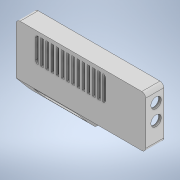
# Autodesk Inventor part: top
Saved by Autodesk Inventor 2021 (Build 250183000, 183)
## iProperties
Created: 2024-09-17
Part Number: top
Material: Generic
Document SubType Name: Modeling
Designer: Toby
Density: 1 g/cm^3
Appearance: Default
Author: Toby
Autodesk Inventor part; units mm, degrees
ref_plane "YZ Plane" through (0, 0, 0) normal (1, 0, 0) x (0, 1, 0)
ref_plane "XZ Plane" through (0, 0, 0) normal (0, 1, 0) x (-1, 0, 0)
ref_plane "XY Plane" through (0, 0, 0) normal (0, 0, 1) x (1, 0, 0)
sketch "Sketch1" plane through (0, 0, 0) normal (0, 0, 1) x (1, 0, 0)
  line L0 (-50, 26) -> (50, 26)
  line L1 (50, 26) -> (50, -26)
  line L2 (50, -26) -> (-50, -26)
  line L3 (-50, -26) -> (-50, 26)
  point P0 (0, 0)
  dimension "d0" = 52
  dimension "d1" = 100
  dimension "d2" = 26
  dimension "d3" = 50
  constraints: 8 end point, 2 parallel, 1 horizontal, 1 perpendicular
  measures "d0" distance of L2.end L0.start
  measures "d1" distance of L0.start L0.end
  measures "d2" distance from line of point (0, 0) L0
  measures "d3" distance from line of point (0, 0) L3
extrude "Extrusion1" add sketch "Sketch1" along normal blind 2
sketch "Sketch4" plane through (0, 0, 2) normal (0, 0, 1) x (1, 0, 0)
  line L0 (50, -26) -> (50, 26) projected
  line L1 (50, -26) -> (13.1, -26)
  line L2 (13.1, -26) -> (13.1, -13.5)
  line L3 (13.1, -13.5) -> (50, -13.5)
  line L4 (50, -13.5) -> (50, -26)
  line L5 (-50, 26) -> (-50, -26) projected
  point P0 (0, 0)
  dimension "d35" = 12.5
  dimension "d36" = 63.1
  constraints: 8 end point, 2 parallel, 1 horizontal, 1 perpendicular
  measures "d35" distance between parallel lines of L1 L3
  measures "d36" distance between parallel lines of L5 L2
extrude "Extrusion3" cut sketch "Sketch4" against normal blind 3
sketch "Sketch5" plane through (0, 0, 2) normal (0, 0, 1) x (1, 0, 0)
  line L0 (-50, -26) -> (13.1, -26) projected
  line L1 (-50, 26) -> (-50, -26) projected
  line L2 (13.1, -13.5) -> (0.673, -26)
  line L3 (0.673, -26) -> (13.1, -26)
  line L4 (13.1, -26) -> (13.1, -13.5) projected
  line L5 (13.1, -13.5) -> (13.1, -26)
  point P0 (0, 0)
  dimension "d39" = 50.673
  constraints: 6 end point, 1 horizontal, 1 point on line, 1 vertical
  measures "d39" distance from line of L1 L2.end
extrude "Extrusion4" cut sketch "Sketch5" against normal blind 3
sketch "Sketch13" plane through (0, 0, 0) normal (0, 0, -1) x (-1, 0, 0)
  line L0 (50, 26) -> (50, -26) projected
  line L1 (-50, 26) -> (50, 26) projected
  line L2 (50, -26) -> (48, -26)
  line L3 (48, -26) -> (48, 26)
  line L4 (48, 26) -> (50, 26)
  line L5 (50, 26) -> (50, -26)
  line L6 (48, 26) -> (-50, 26)
  line L7 (-50, 26) -> (-50, 24)
  line L8 (-50, 24) -> (48, 24)
  line L9 (48, 24) -> (48, 26)
  line L10 (-50, -13.5) -> (-50, 26) projected
  line L11 (-50, -13.5) -> (-48, -13.5)
  line L12 (-48, -13.5) -> (-48, 24)
  line L13 (-48, 24) -> (-50, 24)
  line L14 (-50, 24) -> (-50, -13.5)
  line L15 (6, 24) -> (-9, 24)
  line L16 (-9, 24) -> (-9, 24.8)
  line L17 (-9, 24.8) -> (6, 24.8)
  line L18 (6, 24.8) -> (6, 24)
  point P0 (0, 0)
  dimension "d79" = 2
  dimension "d80" = 2
  dimension "d81" = 2
  dimension "d82" = 1.2
  dimension "d83" = 44
  dimension "d84" = 59
  constraints: 32 end point, 8 parallel, 4 horizontal, 4 perpendicular, 3 point on line, 1 collinear
  measures "d79" distance of L3.end L4.end
  measures "d80" distance between parallel lines of L1 L8
  measures "d81" distance between parallel lines of L10 L12
  measures "d82" distance between parallel lines of L6 L17
  measures "d83" distance between parallel lines of L0 L18
  measures "d84" distance between parallel lines of L0 L16
extrude "Extrusion12" add sketch "Sketch13" along normal blind 12 contours L0 L2 L3 L1 | L3 L8 L18 L17 L16 L7 L1 | L8 L12 L11 L10
sketch "Sketch14" plane through (0, 0, 0) normal (0, 0, -1) x (-1, 0, 0)
  line L0 (48, -26) -> (48, 24) projected
  line L1 (48, -26) -> (37.4, -26)
  line L2 (37.4, -26) -> (37.4, -24)
  line L3 (37.4, -24) -> (48, -24)
  line L4 (48, -24) -> (48, -26)
  line L5 (50, -26) -> (50, 26) projected
  point P0 (0, 0)
  dimension "d87" = 2
  dimension "d88" = 12.6
  constraints: 8 end point, 2 parallel, 1 horizontal, 1 perpendicular
  measures "d87" distance between parallel lines of L1 L3
  measures "d88" distance between parallel lines of L5 L2
extrude "Extrusion13" add sketch "Sketch14" along normal blind 12
fillet "Fillet3" radius 3 4 edges at (-50, -26, -5) (-50, 26, -5) (50, 26, -5) (50, -13.5, -5)
sketch "Sketch16" plane through (0, 0, 0) normal (0, 0, -1) x (-1, 0, 0)
  line L0 (37.4, -26) -> (37.4, -24) projected
  line L1 (37.4, -26) -> (-0.673, -26) projected
  line L2 (37.4, -24) -> (3.6, -24)
  line L3 (3.6, -24) -> (3.6, -26)
  line L4 (3.6, -26) -> (37.4, -26)
  line L5 (37.4, -26) -> (37.4, -24)
  point P0 (0, 0)
  dimension "d95" = 33.8
  constraints: 8 end point, 2 parallel, 1 horizontal, 1 perpendicular, 1 point on line
  measures "d95" distance of L0.end L2.end
extrude "Extrusion15" add sketch "Sketch16" along normal blind 4.4
sketch "Sketch21" plane through (0, 0, 0) normal (0, 0, -1) x (-1, 0, 0)
  line L0 (-13.1, -13.5) -> (-0.673, -26) projected
  line L1 (-13.1, -13.5) -> (-0.673, -26)
  line L2 (3.6, -26) -> (3.6, -24) projected
  line L3 (-0.673, -26) -> (3.6, -26)
  line L4 (3.6, -26) -> (3.6, -24)
  line L5 (3.6, -24) -> (-0.673, -24)
  line L6 (-0.673, -24) -> (-13.1, -11.5)
  line L7 (-13.1, -11.5) -> (-13.1, -13.5)
  point P0 (0, 0)
  dimension "d117" = 2
  dimension "d118" = 2
  constraints: 12 end point, 3 equal length, 3 perpendicular
  measures "d117" distance of L2.start L2.end
  measures "d118" distance of L6.end L0.start
extrude "Extrusion20" add sketch "Sketch21" along normal blind 12
sketch "Sketch22" plane through (0, 0, 0) normal (0, 0, -1) x (-1, 0, 0)
  line L0 (-0.673, -24) -> (-13.1, -11.5) projected
  line L1 (-13.1, -13.5) -> (-47, -13.5) projected
  line L2 (-13.1, -11.5) -> (-47, -11.5)
  line L3 (-47, -11.5) -> (-47, -13.5)
  line L4 (-47, -13.5) -> (-13.1, -13.5)
  line L5 (-13.1, -13.5) -> (-13.1, -11.5)
  arc A0 (-48, -13.3284) -> (-47, -13.5) centre (-47, -10.5) ccw projected
  circle A1 centre (-47, -10.5) radius 3
  circle A2 centre (-47, -10.5) radius 1
  line L6 (-48, 24) -> (-48, -13.3284) projected
  line L7 (-48, -10.5) -> (-48, -13.3284)
  line L8 (-48, -13.3284) -> (-47, -13.5)
  point P0 (0, 0)
  constraints: 12 end point, 2 centre point, 2 coincident, 2 parallel, 2 point on circle, 1 collinear, 1 horizontal, 1 perpendicular, 1 point on line, 1 tangent
extrude "Extrusion21" add sketch "Sketch22" along normal blind 12 contours L1 A1 L2 L5 | L8 L6 A2 L3 | L3 L2 A1 | A0 L8
sketch "Sketch23" plane through (13.1, -13.5, -12) normal (0, -1, 0) x (1, 0, 0)
  line L0 (-63.1, 14) -> (-63.1, 0) projected
  circle A0 centre (6.9, 6.7088) radius 4
  circle A1 centre (25.9, 6.7088) radius 4
  line L1 (34.9, 0) -> (-4.1, 0) projected
  line L2 (2.9, 6.7088) -> (10.9, 6.7088)
  line L3 (10.9, 6.7088) -> (10.9, 0)
  line L4 (10.9, 0) -> (2.9, 0)
  line L5 (2.9, 0) -> (2.9, 6.7088)
  line L6 (21.9, 6.7088) -> (29.9, 6.7088)
  line L7 (29.9, 6.7088) -> (29.9, 0)
  line L8 (29.9, 0) -> (21.9, 0)
  line L9 (21.9, 0) -> (21.9, 6.7088)
  point P0 (-13.1, 12)
  point P1 (21.9, 0)
  point P2 (29.9, 6.7088)
  point P3 (2.9, 0)
  dimension "d125" = 8
  dimension "d126" = 8
  dimension "d123" = 70
  dimension "d124" = 89
  constraints: 16 end point, 4 parallel, 3 point on line, 2 coincident, 2 horizontal, 2 perpendicular, 6 other
  measures "d123" distance from line of L0 point (6.9, 6.709)
  measures "d124" distance from line of L0 point (25.9, 6.709)
extrude "Extrusion22" cut sketch "Sketch23" against normal blind 2
sketch "Sketch24" plane through (50, -10.5, -12) normal (1, 0, 0) x (0, 0, -1)
  line L0 (-14, 0) -> (-14, 33.5) projected
  line L1 (0, 36.5) -> (-14, 36.5) projected
  circle A0 centre (-6, 26.5) radius 4
  circle A1 centre (-6, 14.5) radius 4
  point P0 (-12, 10.5)
  dimension "d129" = 8
  dimension "d130" = 10
  dimension "d131" = 12
  dimension "d132" = 8
  dimension "d133" = 8
  dimension "d134" = 8
  constraints: 2 centre point, 2 coincident
  measures "d129" distance from line of point (-6, 26.5) L0
  measures "d130" distance from line of L1 point (-6, 26.5)
  measures "d131" distance of point (-6, 26.5) point (-6, 14.5)
  measures "d132" distance from line of L0 point (-6, 14.5)
  measures "d133" diameter of A0
  measures "d134" diameter of A1
extrude "Extrusion23" cut sketch "Sketch24" against normal blind 2
sketch "Sketch27" plane through (0, 0, -12) normal (0, 0, -1) x (-1, 0, 0)
  line L0 (50, -23) -> (50, 23) projected
  line L1 (-0.673, -26) -> (47, -26) projected
  line L2 (-0.673, -26) -> (3.6, -26) projected
  line L3 (3.6, -26) -> (37.4, -26) projected
  line L4 (47, 26) -> (-47, 26) projected
  circle A0 centre (-47, 23) radius 2.4
  circle A1 centre (-47, -11) radius 2.4
  circle A2 centre (47, -23) radius 2.4
  circle A3 centre (0, -23) radius 2.4
  circle A4 centre (47, 23) radius 2.4
  point P0 (0, 0)
  point P1 (42.2, -26)
  point P2 (5.6, -26)
  dimension "d144" = 3
  dimension "d145" = 3
  dimension "d146" = 3
  dimension "d147" = 50
  dimension "d148" = 97
  dimension "d149" = 15
  dimension "d150" = 3
  dimension "d151" = 3
  dimension "d152" = 97
  dimension "d153" = 49
  dimension "d154" = 4.8
  dimension "d155" = 4.8
  dimension "d156" = 4.8
  dimension "d157" = 4.8
  dimension "d158" = 4.8
  constraints: 5 centre point, 5 coincident
  measures "d144" distance from line of L0 point (47, -23)
  measures "d145" distance from line of L1 point (47, -23)
  measures "d146" distance from line of L2 point (0, -23)
  measures "d147" distance from line of L0 point (0, -23)
  measures "d148" distance from line of L0 point (-47, -11)
  measures "d149" distance from line of L3 point (-47, -11)
  measures "d150" distance from line of L4 point (47, 23)
  measures "d151" distance from line of L0 point (47, 23)
  measures "d152" distance from line of L0 point (-47, 23)
  measures "d153" distance from line of L3 point (-47, 23)
  measures "d154" diameter of A0
  measures "d155" diameter of A1
  measures "d156" diameter of A2
  measures "d157" diameter of A3
  measures "d158" diameter of A4
extrude "Extrusion26" add sketch "Sketch27" against normal blind 5
sketch "Sketch28" plane through (0, 0, -12) normal (0, 0, -1) x (-1, 0, 0)
  arc A0 (-48, 20.8183) -> (-44.8183, 24) centre (-47, 23) ccw projected
  arc A1 (-44.6527, -11.5) -> (-48, -8.8183) centre (-47, -11) ccw projected
  arc A2 (44.8183, 24) -> (48, 20.8183) centre (47, 23) ccw projected
  arc A3 (48, -20.8183) -> (44.8183, -24) centre (47, -23) ccw projected
  arc A4 (2.1817, -24) -> (-2.311, -22.3524) centre (0, -23) ccw projected
  point P0 (0, 0)
  constraints: 5 coincident
hole "Hole2" at (47, 23, -12) at (47, -11, -12) at (-47, 23, -12) at (-47, -23, -12) at (0, -23, -12) direction (0, 0, 1) diameter 2 depth 4 tip angle 118
chamfer "Chamfer3" distance 2 angle 45 2 edges at (46.4091, 24, -7) (-46.4091, 24, -7)
chamfer "Chamfer4" distance 1 angle 45 3 edges at (45.8263, -11.5, -7) (47.7071, -11.2071, -7) (48, -9.6591, -7)
chamfer "Chamfer5" distance 2 angle 45 4 edges at (-46.4091, -24, -7) (-0.7544, -24, -7) (1.492, -23.1762, -7) (-48, -22.4091, -7)
chamfer "Chamfer6" distance 2 angle 45 1 edges at (-48, 21.4091, -7)
chamfer "Chamfer7" distance 0.8 angle 45 2 edges at (-6, 24, -6) (9, 24, -6)
sketch "Sketch29" plane through (0, 0, 2) normal (0, 0, 1) x (1, 0, 0)
  line L0 (18, 23) -> (18, 4)
  line L1 (-50, 23) -> (-50, -23) projected
  line L2 (47, 26) -> (-47, 26) projected
  line L3 (-35, 23) -> (-33, 23)
  line L4 (-33, 23) -> (-33, 4)
  line L5 (-33, 4) -> (-35, 4)
  line L6 (-35, 4) -> (-35, 23)
  line L7 (-31, 23) -> (-29, 23)
  line L8 (-29, 23) -> (-29, 4)
  line L9 (-29, 4) -> (-31, 4)
  line L10 (-31, 4) -> (-31, 23)
  line L11 (-27, 23) -> (-25, 23)
  line L12 (-25, 23) -> (-25, 4)
  line L13 (-25, 4) -> (-27, 4)
  line L14 (-27, 4) -> (-27, 23)
  line L15 (-23, 23) -> (-21, 23)
  line L16 (-21, 23) -> (-21, 4)
  line L17 (-21, 4) -> (-23, 4)
  line L18 (-23, 4) -> (-23, 23)
  line L19 (-19, 23) -> (-17, 23)
  line L20 (-17, 23) -> (-17, 4)
  line L21 (-17, 4) -> (-19, 4)
  line L22 (-19, 4) -> (-19, 23)
  line L23 (-15, 23) -> (-13, 23)
  line L24 (-13, 23) -> (-13, 4)
  line L25 (-13, 4) -> (-15, 4)
  line L26 (-15, 4) -> (-15, 23)
  line L27 (-11, 23) -> (-9, 23)
  line L28 (-9, 23) -> (-9, 4)
  line L29 (-9, 4) -> (-11, 4)
  line L30 (-11, 4) -> (-11, 23)
  line L31 (-7, 23) -> (-5, 23)
  line L32 (-5, 23) -> (-5, 4)
  line L33 (-5, 4) -> (-7, 4)
  line L34 (-7, 4) -> (-7, 23)
  line L35 (-3, 23) -> (-1, 23)
  line L36 (-1, 23) -> (-1, 4)
  line L37 (-1, 4) -> (-3, 4)
  line L38 (-3, 4) -> (-3, 23)
  line L39 (1, 23) -> (3, 23)
  line L40 (3, 23) -> (3, 4)
  line L41 (3, 4) -> (1, 4)
  line L42 (1, 4) -> (1, 23)
  line L43 (5, 23) -> (7, 23)
  line L44 (7, 23) -> (7, 4)
  line L45 (7, 4) -> (5, 4)
  line L46 (5, 4) -> (5, 23)
  line L47 (9, 23) -> (11, 23)
  line L48 (11, 23) -> (11, 4)
  line L49 (11, 4) -> (9, 4)
  line L50 (9, 4) -> (9, 23)
  line L51 (13, 23) -> (15, 23)
  line L52 (15, 23) -> (15, 4)
  line L53 (15, 4) -> (13, 4)
  line L54 (13, 4) -> (13, 23)
  line L55 (17, 23) -> (19, 23)
  line L56 (19, 23) -> (19, 4)
  line L57 (19, 4) -> (17, 4)
  line L58 (17, 4) -> (17, 23)
  point P0 (0, 0)
  point P1 (-37, 23)
  dimension "d184" = 68
  constraints: 114 end point, 28 parallel, 14 horizontal, 14 perpendicular
  measures "d184" distance between parallel lines of L1 L0
extrude "Extrusion27" cut sketch "Sketch29" against normal blind 2
fillet "Fillet4" radius 2 4 edges at (-35, 23, 1) (-35, 4, 1) (19, 23, 1) (19, 4, 1)
sketch "Sketch30" plane through (-50, -23, -12) normal (-1, 0, 0) x (0, 0, 1)
  line L0 (0, 14.1817) -> (0, 43.8183) projected
  circle A0 centre (0, 25) radius 1
  line L1 (14, 49) -> (0, 49) projected
  point P0 (12, 23)
  point P1 (0, 26)
  point P2 (0, 24)
  dimension "d192" = 2
  dimension "d193" = 24
  constraints: 1 centre point, 1 point on line
  measures "d192" diameter of A0
  measures "d193" distance from line of L1 A0.centre
extrude "Extrusion28" cut sketch "Sketch30" against normal blind 2 contours L0 A0 picked at (0.3333, 25)
sketch "Sketch31" plane through (-50, -23, 2) normal (-1, 0, 0) x (0, 0, 1)
  line L0 (-14, 43.5) -> (-10.5, 43.5)
  line L1 (-10.5, 43.5) -> (-10.5, 33.5)
  line L2 (-10.5, 33.5) -> (-14, 33.5)
  line L3 (-14, 33.5) -> (-14, 43.5)
  line L4 (-14, 0) -> (-14, 24) projected
  line L5 (-14, -3) -> (0, -3) projected
  point P0 (-2, 23)
  dimension "d196" = 36.5
  dimension "d197" = 46.5
  dimension "d198" = 3.5
  constraints: 8 end point, 2 parallel, 1 collinear, 1 horizontal, 1 perpendicular
  measures "d196" distance between parallel lines of L5 L2
  measures "d197" distance between parallel lines of L5 L0
  measures "d198" distance between parallel lines of L3 L1
extrude "Extrusion29" cut sketch "Sketch31" against normal blind 2
sketch "Sketch32" plane through (-50, -23, 2) normal (-1, 0, 0) x (0, 0, 1)
  line L0 (-14, 20) -> (-10.5, 20)
  line L1 (-10.5, 20) -> (-10.5, 9.5)
  line L2 (-10.5, 9.5) -> (-14, 9.5)
  line L3 (-14, 9.5) -> (-14, 20)
  line L4 (-14, -3) -> (0, -3) projected
  line L5 (-14, 0) -> (-14, 24) projected
  point P0 (-2, 23)
  dimension "d201" = 12.5
  dimension "d202" = 23
  dimension "d203" = 3.5
  constraints: 8 end point, 2 parallel, 1 collinear, 1 horizontal, 1 perpendicular
  measures "d201" distance between parallel lines of L4 L2
  measures "d202" distance between parallel lines of L4 L0
  measures "d203" distance between parallel lines of L3 L1
extrude "Extrusion30" cut sketch "Sketch32" against normal blind 2
fillet "Fillet5" radius 1 4 edges at (-49, 20.5, -8.5) (-49, 10.5, -8.5) (-49, -13.5, -8.5) (-49, -3, -8.5)
sketch "Sketch36" plane through (0, 0, 2) normal (0, 0, 1) x (1, 0, 0)
  line L0 (-47, -26) -> (0.673, -26) projected
  line L1 (-42.4, -26) -> (-3.6, -26)
  line L2 (-3.6, -26) -> (-3.6, -16)
  line L3 (-3.6, -16) -> (-42.4, -16)
  line L4 (-42.4, -16) -> (-42.4, -26)
  line L5 (-50, 23) -> (-50, -23) projected
  point P0 (0, 0)
  point P1 (-3.6, -26)
  dimension "d217" = 7.6
  dimension "d218" = 10
  dimension "d219" = 46.4
  constraints: 8 end point, 2 parallel, 1 horizontal, 1 perpendicular, 1 point on line
  measures "d217" distance between parallel lines of L5 L4
  measures "d218" distance between parallel lines of L0 L3
  measures "d219" distance between parallel lines of L5 L2
extrude "Extrusion34" cut sketch "Sketch36" against normal blind 20
sketch "Sketch37" plane through (-50, -23, 2) normal (-1, 0, 0) x (0, 0, 1)
  line L0 (0, 9.5) -> (-14, 9.5) projected
  line L1 (0, 9.5) -> (-10.4887, -3)
  line L2 (0, 9.5) -> (16.3176, 9.5) construction
  line L3 (-10.4887, -3) -> (0, -3)
  line L4 (0, -3) -> (-14, -3) projected
  line L5 (0, -3) -> (0, 9.5)
  line L6 (0, -3) -> (0, 9.5) projected
  line L7 (0, 46) -> (0, 0) projected
  point P0 (-2, 23)
  dimension "d222" = 130
  constraints: 8 end point, 3 collinear, 1 equal length, 1 horizontal, 1 point on line
  measures "d222" angle of L1 L2
extrude "Extrusion35" cut sketch "Sketch37" against normal blind 67
sketch "Sketch38" plane through (-50, -13.5, 2) normal (0, -0.6427876, 0.7660444) x (1, 0, 0)
  line L0 (2, -3.1114) -> (2, -10.8901) projected
  line L1 (2, -3.1114) -> (2, -10.8901)
  line L2 (7.6, -16.3176) -> (3, -16.3176) projected
  line L3 (2, -10.8901) -> (3, -16.3176)
  line L4 (3, -16.3176) -> (50.673, -16.3176)
  ellipse E0 centre (50, -16.2764) end of major axis (49, -16.2764) minor radius 0.766 projected
  line L5 (63.1, 0) -> (50.673, -16.3176) projected
  line L6 (50.673, -16.3176) -> (63.1, 0)
  line L7 (63.1, 0) -> (2, 0)
  line L8 (0, 0) -> (63.1, 0) projected
  line L9 (58.7421, -3.1114) -> (2, -3.1114) projected
  line L10 (2, -3.1114) -> (2, 0)
  line L11 (2, -5.9832) -> (2, 0.5282) projected
  point P0 (50, 9.056)
  point P1 (7.6, -16.3176)
  point P2 (49.0014, -16.3176)
  point P3 (50.9254, -15.9862)
  constraints: 12 end point, 2 collinear, 2 point on line, 1 horizontal, 1 vertical, 1 other
extrude "Extrusion36" add sketch "Sketch38" against normal blind 1.2 contours L10 L7 L5 E0 L4 L2 L3 L0
sketch "Sketch39" plane through (-47, -26, -12) normal (0, -1, 0) x (1, 0, 0)
  line L0 (4.6, 0) -> (4.6, 3.5113) projected
  line L1 (43.4, 0) -> (43.4, 3.623) projected
  line L2 (4.6, 3.5113) -> (43.4, 3.5113)
  line L3 (43.4, 3.5113) -> (43.4, 0)
  line L4 (43.4, 0) -> (4.6, 0)
  line L5 (4.6, 0) -> (4.6, 3.5113)
  point P0 (47, 12)
  point P1 (43.4, 3.5113)
  constraints: 8 end point, 2 parallel, 1 horizontal, 1 perpendicular
extrude "Extrusion37" add sketch "Sketch39" against normal blind 1.2
fillet "Fillet6" radius 3 1 edges at (0.673, -26, -10.2444)
sketch "Sketch40" plane through (-50, -13.5, 2) normal (0, -0.6427876, 0.7660444) x (1, 0, 0)
  line L0 (12, -2.6813) -> (45.2, -2.6813)
  line L1 (45.2, -2.6813) -> (45.2, -14.9813)
  line L2 (45.2, -14.9813) -> (12, -14.9813)
  line L3 (12, -14.9813) -> (12, -2.6813)
  line L4 (60.5981, -1.6813) -> (2, -1.6813) projected
  line L5 (2, -1.6813) -> (2, -10.5602) projected
  point P0 (50, 9.056)
  dimension "d230" = 12.3
  dimension "d231" = 33.2
  dimension "d232" = 1
  dimension "d233" = 10
  constraints: 8 end point, 2 parallel, 1 horizontal, 1 perpendicular
  measures "d230" distance between parallel lines of L2 L0
  measures "d231" distance of L0.start L0.end
  measures "d232" distance between parallel lines of L4 L0
  measures "d233" distance between parallel lines of L5 L3
extrude "Extrusion38" cut sketch "Sketch40" against normal blind 1.2
sketch "Sketch41" plane through (0, 0, -12) normal (0, 0, -1) x (-1, 0, 0)
  line L0 (-48, -8.8183) -> (-48, 20.8183) projected
  line L1 (-48, 11.5) -> (-48.8, 11.5)
  line L2 (-48.8, 11.5) -> (-48.8, -8.5)
  line L3 (-48.8, -8.5) -> (-48, -8.5)
  line L4 (-48, -8.5) -> (-48, 11.5)
  line L5 (-50, 23) -> (-50, -10.5) projected
  line L6 (-47, -13.5) -> (-43, -13.5) projected
  point P0 (0, 0)
  dimension "d236" = 1.2
  dimension "d237" = 5
  dimension "d238" = 20
  constraints: 8 end point, 2 parallel, 1 horizontal, 1 perpendicular, 1 point on line
  measures "d236" distance between parallel lines of L5 L2
  measures "d237" distance between parallel lines of L6 L3
  measures "d238" distance from line of L3.end L1
extrude "Extrusion39" cut sketch "Sketch41" against normal blind 1.5
chamfer "Chamfer8" distance 1.5 angle 45 2 edges at (48.4, -8.5, -10.5) (48.4, 11.5, -12)
body "Solid1"
